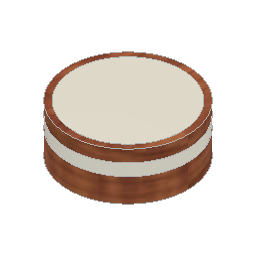
LuminaBreath (Autodesk Fusion 360 design; units mm, degrees)
Autodesk Fusion 360 part; units mm, degrees
sketch "Sketch1" plane through (0, 0, 0) normal (0, 1, 0) x (1, 0, 0) in component "TopInset"
  circle A0 centre (0, 0) radius 45
  dimension "d1" = 90
  constraint coincident A0.centre origin
  measures "d1" diameter of A0
extrude "Extrude1" add sketch "Sketch1" along normal blind 3 makes body 1 in component "TopInset"
sketch "Sketch1 (2)" plane through (0, 3, 0) normal (0, 1, 0) x (-1, 0, 0) in component "MiddleRing"
  circle A0 centre (0, 0) radius 45
  circle A1 centre (0, 0) radius 40
  circle A2 centre (0, 0) radius 50
  dimension "d4" = 80
  dimension "d5" = 100
  constraint coincident A0.centre A1.centre
  constraint concentric A1 A2
  measures "d4" diameter of A1
  measures "d5" diameter of A2
extrude "Extrude1'" add sketch "Sketch1 (2)" along normal blind 10 separate body contours A0 | A2 makes body 2 in component "MiddleRing"
copy_body "CopyPasteBodies1" bodies 2 makes body 3
move_body "Move1" bodies 3 to x (1, 0, 0) y (0, 1, 0) z (0, 0, 1) at (0, 36, 0)
move_face "MoveFace1" to x (1, 0, 0) y (0, 1, 0) z (0, 0, 1) at (0, -49, 0) 1 faces at (49.9378, 42.3333, 2.4923) on bodies 3
move_face "MoveFace2" to x (1, 0, 0) y (0, 1, 0) z (0, 0, 1) at (0, -49, 0) 1 faces at (49.9378, 42.3333, 2.4923) on bodies 3
copy_body "CutPasteBodies1" bodies 3 removing the originals makes body 4 in component "TopRing"
sketch "Sketch1 (3)" plane through (0, 0, 0) normal (1, 0, 0) x (0, 0, -1) in component "TopRing"
sketch "Sketch2" plane through (0, 0, 0) normal (0, 0, 1) x (1, 0, 0) in component "TopRing"
combine "Combine1" operation cut target body 4 tool bodies 1 body 1 seen with x (1, 0, 0) y (0, 1, 0) z (0, 0, 1) at (0, 46, 0) keep tools in component "TopRing"
extrude "Extrude1''" add 1 faces at (-46.3316, 3, -4.4713) along direction (0, -1, 0) blind 10 separate body on bodies 2 makes body 5 in component "BottomRing"
surface "SurfacePatch1" add patch along 1 edges at (37.2931, -7, -14.4646) separate body on bodies 5 makes body 6 in component "BottomRing"
extrude "Extrude2" add 1 faces at (-9.4847, -7, -14.2223) along direction (0, -1, 0) blind 10 separate body on bodies 6 makes body 7 in component "BottomRing"
extrude "Extrude3" add 1 faces at (-46.3316, -7, -4.4713) along direction (0, -1, 0) blind 10 on bodies 5 bodies 5 7 in component "BottomRing"
component "TopInset" placed x (1, 0, 0) y (0, 1, 0) z (0, 0, 1) at (0, 100, 0)
component "MiddleRing" placed x (1, 0, 0) y (0, 1, 0) z (0, 0, 1) at (0, 80, 0)
component "TopRing" placed x (1, 0, 0) y (0, 1, 0) z (0, 0, 1) at (0, 54, 0)
component "BottomRing" placed x (1, 0, 0) y (0, 1, 0) z (0, 0, 1) at (0, 80, 0)
